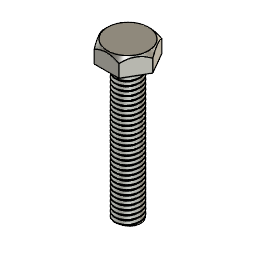
M6_32_mm_hex_bolt (Autodesk Fusion 360 design; units mm, degrees)
part number: 2026-04-25-09-17-42-437
Autodesk Fusion 360 part; units mm, degrees
sketch "Diameter" plane through (0, 0, 0) normal (0, 0, 1) x (1, 0, 0)
  circle A0 centre (0, 0) radius 3
  dimension "d2" = 6
  constraint coincident A0.centre origin
  measures "d2" diameter of A0
extrude "Extrude1" add sketch "Diameter" along normal blind 32
sketch "Head" plane through (0, 0, 32) normal (0, 0, 1) x (-1, 0, 0)
  circle A0 centre (0, 0) radius 3
  line L0 (2.8868, -5) -> (5.7735, 0)
  line L1 (5.7735, 0) -> (2.8868, 5)
  line L2 (2.8868, 5) -> (-2.8868, 5)
  line L3 (-2.8868, 5) -> (-5.7735, 0)
  line L4 (-5.7735, 0) -> (-2.8868, -5)
  line L5 (-2.8868, -5) -> (2.8868, -5)
  dimension "d10" = 10
  constraint coincident A0.centre origin
  measures "d10" distance of L2 L5
extrude "Extrude2" add sketch "Head" along normal blind 4 contours A0 | L0 L1 L2 L3 L4 L5
thread "Thread1" "ISO Metric profile 6.0 M6x1 M6x1 6g" major diameter 5.884 minor diameter 4.7435 pitch 1 angle 60 modelled right hand crest width 0.1444 on face at (2.9963, -0.1495, 21.3333) crest through (2.942, 0, -0.25)
sketch "Head fillet" plane through (0, 0, 0) normal (0, 1, 0) x (1, 0, 0)
  line L0 (2.8868, -32) -> (5.7735, -32)
  line L1 (5.7735, -32) -> (5.7735, -36)
  line L2 (5.7735, -36) -> (2.8868, -36)
  line L3 (2.8868, -36) -> (2.8868, -32)
  line L4 (-5.7735, -32) -> (-2.8868, -32)
  line L5 (-2.8868, -32) -> (-2.8868, -36)
  line L6 (-2.8868, -36) -> (-5.7735, -36)
  line L7 (-5.7735, -36) -> (-5.7735, -32)
  line L8 (-2.8868, -32) -> (2.8868, -32)
  line L9 (2.8868, -32) -> (2.8868, -36)
  line L10 (2.8868, -36) -> (-2.8868, -36)
  line L11 (-2.8868, -36) -> (-2.8868, -32)
  line L12 (5.7735, -36) -> (4.7735, -36)
  line L13 (5.7735, -36) -> (5.7735, -35)
  line L14 (4.7735, -36) -> (5.7735, -35)
  dimension "d14" = 1
  dimension "d15" = 1
  constraint coincident L1.end L2.start
  constraint perpendicular L1 L12
  constraint perpendicular L2 L13
  measures "d14" distance of L1.end L12.end
  measures "d15" distance of L1.end L13.end
revolve "Revolve1" cut sketch "Head fillet" angle 360 about axis through (0, 0, 1.75) along (0, 0, 1) contours L1 L2 L12 L13 L14
equation "diameter = 6 mm" comment "An M6 hex bolt has a diameter of 6 mm."
equation "d2 = diameter"
equation "thread_height = 32 mm" comment "The length of the M6 hex bolt (excluding the head)."
equation "d4 = thread_height"
equation "head_height = 4 mm" comment "An M6 hex bolt has a head thickness of 4 mm."
equation "width_across_flats = 10 mm" comment "An M6 hex bolt has a width across the flats of 10 mm."
equation "d10 = width_across_flats"
equation "d11 = head_height"
equation "chamfer_side_length = 1 mm" comment "Chamfer on the top of the hex bolt head."
equation "d14 = chamfer_side_length"
equation "d15 = chamfer_side_length"
named bodies: "M6 Thread"
